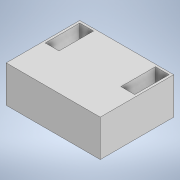
# Autodesk Inventor part: chassi1
Saved by Autodesk Inventor 2020 (Build 240168000, 168)
## iProperties
Created: 2020-04-18
Part Number: chassi1
Material: Genérico
Document SubType Name: Modeling
Designer: eduardoADM
Density: 1 g/cm^3
Appearance: Padrão
Author: eduardoADM
Autodesk Inventor part; units mm, degrees
ref_plane "YZ Plane" through (0, 0, 0) normal (1, 0, 0) x (0, 1, 0)
ref_plane "XZ Plane" through (0, 0, 0) normal (0, 1, 0) x (-1, 0, 0)
ref_plane "XY Plane" through (0, 0, 0) normal (0, 0, 1) x (1, 0, 0)
sketch "Esboço3" plane through (0, 0, 0) normal (0, 0, 1) x (1, 0, 0)
  line L0 (0, 0) -> (204.6, 0)
  line L1 (204.6, 0) -> (204.6, 80)
  line L2 (204.6, 80) -> (0, 80)
  line L3 (0, 80) -> (0, 0)
  dimension "d4" = 204.6
  dimension "d5" = 80
  constraints: 8 end point, 2 parallel, 1 horizontal, 1 perpendicular
  measures "d4" distance of L2.end L1.end
  measures "d5" distance of L1.end L0.end
extrude "Extrusão2" add sketch "Esboço3" along normal blind 160
sketch "Esboço7" plane through (0, 80, 0) normal (0, 1, 0) x (1, 0, 0)
  line L0 (0, 0) -> (5, 0)
  line L1 (0, 0) -> (204.6, 0) projected
  line L2 (5, -5) -> (5, -80)
  line L3 (5, -80) -> (35, -80)
  line L4 (5, -5) -> (35, -5)
  line L5 (35, -5) -> (35, -80)
  line L6 (35, -80) -> (5, -80)
  line L7 (5, -80) -> (5, -5)
  line L8 (204.6, 0) -> (204.6, -160) projected
  line L9 (199.6, -5) -> (199.6, -80)
  line L10 (199.6, -80) -> (169.6, -80)
  line L11 (199.6, -5) -> (169.6, -5)
  line L12 (169.6, -5) -> (169.6, -80)
  line L13 (169.6, -80) -> (199.6, -80)
  line L14 (199.6, -80) -> (199.6, -5)
  constraints: 26 end point, 4 parallel, 4 perpendicular, 2 horizontal, 1 point on line
extrude "Extrusão3" cut sketch "Esboço7" against normal through all
